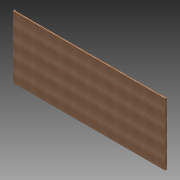
# Autodesk Inventor part: Base
Saved by Autodesk Inventor 2014 SP1 (Build 180222100, 222)
## iProperties
Created: 2015-03-28
Part Number: Base
Material: Wood (Birch)
Document SubType Name: Modeling
Designer: tuleu
Density: 0.55 g/cm^3
Appearance: Birch - Natural Polished
Author: tuleu
Autodesk Inventor part; units mm, degrees
ref_plane "YZ Plane" through (0, 0, 0) normal (1, 0, 0) x (0, 1, 0)
ref_plane "XZ Plane" through (0, 0, 0) normal (0, 1, 0) x (-1, 0, 0)
ref_plane "XY Plane" through (0, 0, 0) normal (0, 0, 1) x (1, 0, 0)
sketch "Sketch1" plane through (0, 0, 0) normal (0, 1, 0) x (-1, 0, 0)
  line L0 (1400, 575) -> (-1400, 575)
  line L1 (-1400, 575) -> (-1400, -575)
  line L2 (-1400, -575) -> (1400, -575)
  line L3 (1400, -575) -> (1400, 575)
  line L4 (0, -575) -> (0, 575)
  line L5 (-1400, 0) -> (1400, 0)
  point P0 (0, 0)
  dimension "d0" = 2800
  dimension "d1" = 1150
  constraints: 12 end point, 6 midpoint, 2 parallel, 1 horizontal, 1 perpendicular
  measures "d0" distance of L1.end L2.end
  measures "d1" distance of L2.end L0.start
extrude "Extrusion1" add sketch "Sketch1" along normal blind 19
sketch "Sketch2" plane through (0, 19, 0) normal (0, 1, 0) x (1, 0, 0)
  line L0 (1400, 575) -> (-1400, 575) projected
  line L1 (-1400, 575) -> (-1400, -575) projected
  line L2 (-1400, -575) -> (1400, -575) projected
  line L3 (1400, -575) -> (1400, 575) projected
  line L4 (-1385, -575) -> (-1385, 475)
  line L5 (-1385, 475) -> (1385, 475)
  line L6 (1385, 475) -> (1385, -575)
  line L7 (-1385, -575) -> (-1400, -575)
  line L8 (-1400, 575) -> (-1400, -575)
  line L9 (-1400, 575) -> (1400, 575)
  line L10 (1400, 575) -> (1400, -575)
  line L11 (1400, -575) -> (1385, -575)
  point P0 (0, 0)
  dimension "d4" = 15
  dimension "d5" = 15
  dimension "d6" = 100
  constraints: 16 end point, 5 perpendicular, 2 collinear, 2 point on line, 1 parallel
  measures "d4" distance between parallel lines of L1 L4
  measures "d5" distance between parallel lines of L3 L6
  measures "d6" distance between parallel lines of L0 L5
extrude "Extrusion2" add sketch "Sketch2" along normal blind 19 contours L3 L2 L6 L5 L4 L1 L0
body "Solid1"
